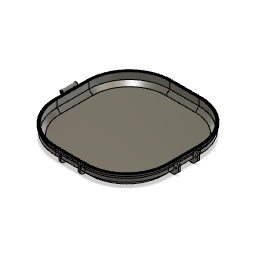
BoxFilament_Remix (Autodesk Fusion 360 archive; units mm, degrees)
design "BoxFilament_Lid_VII_v6"
Autodesk Fusion 360 part; units mm, degrees
sketch "Sketch1" plane through (0, 0, 0) normal (0, 1, 0) x (1, 0, 0)
  line L0 (28, -100.5) -> (-28, -100.5)
  line L1 (-98, -30.5) -> (-98, 30.5)
  line L2 (-28, 100.5) -> (28, 100.5)
  line L3 (98, 30.5) -> (98, -30.5)
  line L4 (98, -100.5) -> (-98, 100.5) construction
  line L5 (-98, -100.5) -> (98, 100.5) construction
  arc A0 (-28, 100.5) -> (-98, 30.5) centre (-28, 30.5) ccw
  arc A1 (98, 30.5) -> (28, 100.5) centre (28, 30.5) ccw
  arc A2 (28, -100.5) -> (98, -30.5) centre (28, -30.5) ccw
  arc A3 (-98, -30.5) -> (-28, -100.5) centre (-28, -30.5) ccw
  line L6 (15, 100.5) -> (15, -100.5)
  line L7 (-15, 100.5) -> (-15, -100.5)
  line L8 (-98, 15) -> (98, 15)
  line L9 (-98, -15) -> (98, -15)
  line L10 (0, 0) -> (0, -36) construction
  circle A4 centre (0, -36) radius 1.85
  circle A5 centre (36, 0) radius 1.85
  circle A6 centre (0, 36) radius 1.85
  circle A7 centre (-36, 0) radius 1.85
  dimension "d6" = 201
  dimension "d7" = 196
  dimension "d8" = 70
  dimension "d9" = 70
  dimension "d10" = 70
  dimension "d11" = 70
  dimension "d150" = 15
  dimension "d151" = 15
  dimension "d176" = 15
  dimension "d177" = 15
  dimension "d218" = 36
  dimension "d219" = 3.7
  dimension "d221" = 360
  constraint horizontal L0
  constraint perpendicular L0 L1
  constraint parallel L0 L2
  constraint parallel L1 L3
  constraint coincident L4 L10.start
  constraint coincident L5 L10.start
  constraint coincident L10.start origin
  constraint coincident L4.end L2
  constraint coincident L4.end L1
  constraint tangent L2 A0
  constraint tangent L1 A0
  constraint coincident L5.end L2
  constraint coincident L5.end L3
  constraint tangent L2 A1
  constraint tangent L3 A1
  constraint coincident L4.start L3
  constraint coincident L4.start L0
  constraint tangent L3 A2
  constraint tangent L0 A2
  constraint coincident L5.start L0
  constraint coincident L5.start L1
  constraint tangent L0 A3
  constraint tangent L1 A3
  constraint coincident L2 L6.start
  constraint coincident L0 L6.end
  constraint vertical L6
  constraint coincident L2 L7.start
  constraint coincident L0 L7.end
  constraint vertical L7
  constraint coincident L1 L8.start
  constraint coincident L3 L8.end
  constraint coincident L1 L9.start
  constraint coincident L3 L9.end
  constraint horizontal L8
  constraint horizontal L9
  constraint vertical L10
  constraint coincident L10.end A4.centre
  measures "d6" distance of L0 L2
  measures "d7" distance of L1 L3
  measures "d8" radius of A0
  measures "d9" radius of A1
  measures "d10" radius of A2
  measures "d11" radius of A3
  measures "d150" distance of L10.start L7
  measures "d151" distance of L10.start L6
  measures "d176" distance of L10.start L8
  measures "d177" distance of L10.start L9
  measures "d218" distance of L10.start L10.end
  measures "d219" diameter of A4
sketch "Sketch2" plane through (0, 0, 0) normal (0, 0, 1) x (1, 0, 0)
  line L0 (0, 0) -> (98, 0)
  line L1 (98, 0) -> (98, 2.4)
  line L2 (105, 9.4) -> (105, 22.4)
  line L3 (105, 22.4) -> (106.23, 22.4)
  line L4 (106.23, 22.4) -> (106.23, 20.4)
  line L5 (106.23, 20.4) -> (108.03, 20.4)
  line L6 (108.03, 20.4) -> (108.03, 22.4)
  line L7 (108.03, 22.4) -> (109.26, 22.4)
  line L8 (109.26, 22.4) -> (109.26, 19.4)
  line L9 (108.1865, 0) -> (98, 0)
  line L10 (109.26, 19.4) -> (107.4, 19.4)
  line L11 (107.4, 19.4) -> (107.4, 15)
  line L12 (107.4, 15) -> (107.4, 8.4059)
  line L13 (107.4, 15) -> (109.26, 19.4)
  line L14 (105, 9.4) -> (98, 2.4)
  line L15 (98.9941, 0) -> (107.4, 8.4059)
  line L16 (108.1865, 0) -> (116.26, 8.0735)
  line L17 (109.26, 22.4) -> (111.26, 22.4)
  line L18 (116.26, 17.4) -> (116.26, 8.0735)
  arc A0 (116.26, 17.4) -> (111.26, 22.4) centre (111.26, 17.4) ccw
  circle A1 centre (111.76, 12.4) radius 1.425
  line L19 (0, 0) -> (0, 60)
  line L20 (-116.26, 17.4) -> (-116.26, 8.0735)
  line L21 (-106.23, 22.4) -> (-106.23, 20.4)
  line L22 (-107.4, 15) -> (-109.26, 19.4)
  line L23 (-105, 9.4) -> (-105, 22.4)
  line L24 (-98, 0) -> (-98, 2.4)
  line L25 (-106.23, 20.4) -> (-108.03, 20.4)
  line L26 (-98.9941, 0) -> (-107.4, 8.4059)
  line L27 (-107.4, 15) -> (-107.4, 8.4059)
  line L28 (-105, 9.4) -> (-98, 2.4)
  line L29 (-109.26, 22.4) -> (-109.26, 19.4)
  line L30 (-108.1865, 0) -> (-116.26, 8.0735)
  line L31 (-107.4, 19.4) -> (-107.4, 15)
  line L32 (-108.03, 22.4) -> (-109.26, 22.4)
  line L33 (-108.03, 20.4) -> (-108.03, 22.4)
  line L34 (-108.1865, 0) -> (-98, 0)
  line L35 (-109.26, 19.4) -> (-107.4, 19.4)
  line L36 (-105, 22.4) -> (-106.23, 22.4)
  line L37 (107.4, 19.4) -> (105, 19.4)
  line L38 (-107.4, 19.4) -> (-105, 19.4)
  circle A2 centre (-112.86, 22.4) radius 1.425
  circle A3 centre (-112.86, 22.4) radius 3.4
  line L39 (-116.26, 22.4) -> (-116.26, 17.4)
  line L40 (-109.26, 22.4) -> (-109.46, 22.4)
  line L41 (-115.2642, 19.9958) -> (-105, 9.7317)
  line L42 (-115.2642, 19.9958) -> (-39.091, 19.9958) construction
  line L43 (-109.26, 22.4) -> (-112.86, 22.4)
  line L44 (106.23, 22.4) -> (108.03, 22.4)
  line L45 (106.38, 22.4) -> (106.38, 20.4)
  line L46 (107.88, 22.4) -> (107.88, 20.4)
  line L47 (107.13, 22.4) -> (107.13, 23.3002)
  line L48 (106.38, 22.4) -> (107.13, 23.3002)
  line L49 (107.13, 23.3002) -> (107.88, 22.4)
  line L50 (107.13, 23.3002) -> (107.33, 23.3002)
  line L51 (107.33, 23.3002) -> (107.33, 23.0602)
  line L52 (107.13, 23.3002) -> (106.93, 23.3002)
  line L53 (106.93, 23.3002) -> (106.93, 23.0602)
  point P0 (116.26, 22.4)
  point P1 (-116.26, 22.4)
  dimension "d12" = 98
  dimension "d13" = 2.4
  dimension "d15" = 1.23
  dimension "d16" = 2
  dimension "d17" = 1.8
  dimension "d18" = 2
  dimension "d20" = 3
  dimension "d23" = 4.4
  dimension "d26" = 2.4
  dimension "d27" = 7
  dimension "d28" = 7
  dimension "d29" = 22.4
  dimension "d30" = 6.5
  dimension "d61" = 7
  dimension "d62" = 5
  dimension "d63" = 2.85
  dimension "d64" = 10
  dimension "d65" = 4.5
  dimension "d129" = 1.23
  dimension "d131" = 2.4
  dimension "d137" = 2.85
  dimension "d138" = 3.6
  dimension "d139" = 6.8
  dimension "d140" = 45
  dimension "d248" = 0.15
  dimension "d249" = 0.15
  dimension "d250" = 79.6
  dimension "d251" = 0.24
  dimension "d252" = 0.24
  constraint coincident L0.start L19.start
  constraint horizontal L0
  constraint perpendicular L0 L1
  constraint perpendicular L2 L3
  constraint perpendicular L3 L4
  constraint perpendicular L4 L5
  constraint perpendicular L5 L6
  constraint perpendicular L6 L7
  constraint perpendicular L7 L8
  constraint perpendicular L1 L9
  constraint perpendicular L8 L10
  constraint perpendicular L10 L11
  constraint perpendicular L9 L12
  constraint coincident L9 L15.start
  constraint vertical L2
  constraint perpendicular L8 L17
  constraint perpendicular L7 L18
  constraint coincident P0 L17
  constraint coincident P0 L18
  constraint tangent L17 A0
  constraint tangent L18 A0
  constraint perpendicular L0 L19
  constraint symmetric L0.end L19 L24.start
  constraint symmetric L1.end L19 L24.end
  constraint symmetric L2.end L19 L23.end
  constraint symmetric L3.end L19 L21.start
  constraint symmetric L4.end L19 L21.end
  constraint symmetric L5.end L19 L25.end
  constraint symmetric L6.end L19 L32.start
  constraint symmetric L7.end L19 L29.start
  constraint symmetric L8.end L19 L22.end
  constraint symmetric L10.end L19 L31.start
  constraint symmetric L11.end L19 L22.start
  constraint symmetric L2.start L19 L23.start
  constraint symmetric L15.start L19 L26.start
  constraint symmetric L12.end L19 L26.end
  constraint symmetric L9.start L19 L30.start
  constraint symmetric P0 L19 P1
  constraint symmetric L16.end L19 L20.end
  constraint symmetric L18.start L19 L20.start
  constraint coincident L2 L37.end
  constraint perpendicular L2 L37
  constraint coincident L23 L38.end
  constraint perpendicular L23 L38
  constraint concentric A2 A3
  constraint coincident P1 L39.start
  constraint coincident A3 L40.end
  constraint horizontal L42
  constraint coincident A3 L41.start
  constraint tangent A3 L41
  constraint coincident L23 L41.end
  constraint horizontal L40
  constraint coincident A2.centre A3.centre
  constraint perpendicular L29 L43
  constraint coincident L44 L45.start
  constraint coincident L5 L45.end
  constraint perpendicular L5 L45
  constraint coincident L44 L46.start
  constraint coincident L5 L46.end
  constraint perpendicular L5 L46
  constraint midpoint L44 L47.start
  constraint perpendicular L44 L47
  constraint perpendicular L47 L50
  constraint coincident L49 L51.end
  constraint perpendicular L50 L51
  constraint perpendicular L47 L52
  constraint coincident L48 L53.end
  constraint perpendicular L52 L53
  measures "d12" distance of L0.start L0.end
  measures "d13" distance of L0.end L1.end
  measures "d15" distance of L2.end L3.end
  measures "d16" distance of L3.end L4.end
  measures "d17" distance of L4.end L5.end
  measures "d18" distance of L5.end L6.end
  measures "d20" distance of L7.end L8.end
  measures "d23" distance of L10.end L11.end
  measures "d26" distance of L14 L15
  measures "d27" vertical distance of L1.end L2.start
  measures "d28" horizontal distance of L1.end L2.start
  measures "d29" distance of L0.end L7
  measures "d30" distance of L15 L16
  measures "d61" distance of L7.end P0
  measures "d62" radius of A0
  measures "d63" diameter of A1
  measures "d64" distance of L17 A1.centre
  measures "d65" distance of L18 A1.centre
  measures "d129" distance of L6 L8
  measures "d131" distance of L2 L12
  measures "d137" diameter of A2
  measures "d138" distance of L29.start A2.centre
  measures "d139" diameter of A3
  measures "d140" angle of L41 L42
  measures "d248" distance of L6 L46
  measures "d249" distance of L4 L45
  measures "d250" angle of L48 L49
  measures "d251" distance of L50.end L51.end
  measures "d252" distance of L52.end L53.end
extrude "Extrude1" add sketch "Sketch1" along normal blind 2.4 contours L0 L3 A2 L6 L9 | L0 L6 L7 L9 | L0 L1 A3 L7 L9 | L6 L7 L8 L9 | L3 L6 L8 L9 | L1 L7 L8 L9 | L2 L6 L7 L8 | L2 L3 A1 L6 L8 | L1 L2 A0 L7 L8 | A4 | A5 | A6 | A7 makes body 1
sweep "Sweep1" add profiles "Sketch2" path "Sketch1" along A2 L0 A3 L1 A0 L2 A1 L3 section 1 contours L1 L2 L9 L11 L12 L14 L15 L37 | L2 L3 L4 L5 L6 L7 L8 L10 L37 | L10 L11 L13 | L4 L5 L44 L45 | L44 L47 L48 | L5 L44 L45 L46 | L5 L6 L44 L46 | L44 L47 L49 | L48 L52 L53 | L49 L50 L51 bodies 1
ref_plane "WorkPlane2" through (-18.4, 0, 0) normal (1, 0, 0) x (0, 1, 0)
sketch "Sketch4" plane through (-18.4, 0, 0) normal (1, 0, 0) x (0, 0, -1)
  line L0 (0, 0) -> (-100.5, 0)
  line L1 (-100.5, 0) -> (-100.5, 2.4)
  line L2 (-100.5, 2.4) -> (-107.5, 2.4)
  line L3 (-107.5, 2.4) -> (-107.5, 9.4)
  line L4 (-107.5, 9.4) -> (-100.5, 2.4)
  line L5 (-107.5, 2.4) -> (-107.5, 5)
  line L6 (-107.5, 2.4) -> (-107.5, 19.4)
  line L7 (-107.5, 19.4) -> (-111.76, 19.4)
  line L8 (-111.76, 19.4) -> (-111.76, 4.4676)
  line L9 (-107.2924, 0) -> (-100.5, 0)
  line L10 (-107.2924, 0) -> (-111.76, 4.4676)
  line L11 (0, 0) -> (0, 70)
  line L12 (107.2924, 0) -> (111.76, 4.4676)
  line L13 (107.2924, 0) -> (100.5, 0)
  line L14 (107.5, 2.4) -> (107.5, 5)
  line L15 (107.5, 2.4) -> (107.5, 19.4)
  line L16 (107.5, 9.4) -> (100.5, 2.4)
  line L17 (107.5, 2.4) -> (107.5, 9.4)
  line L18 (107.5, 19.4) -> (111.76, 19.4)
  line L19 (111.76, 19.4) -> (111.76, 4.4676)
  line L20 (100.5, 0) -> (100.5, 2.4)
  line L21 (100.5, 2.4) -> (107.5, 2.4)
  dimension "d47" = 100.5
  dimension "d48" = 2.4
  dimension "d49" = 7
  dimension "d50" = 7
  dimension "d52" = 4.26
  dimension "d53" = 6.5
  dimension "d56" = 19.4
  constraint coincident L0.start L11.start
  constraint horizontal L0
  constraint perpendicular L0 L1
  constraint perpendicular L1 L2
  constraint perpendicular L2 L3
  constraint coincident L3 L5.end
  constraint perpendicular L2 L6
  constraint perpendicular L6 L7
  constraint perpendicular L7 L8
  constraint perpendicular L1 L9
  constraint perpendicular L0 L11
  constraint symmetric L0.end L11 L13.end
  constraint symmetric L1.end L11 L16.end
  constraint symmetric L2.end L11 L14.start
  constraint symmetric L3.end L11 L16.start
  constraint symmetric L5.end L11 L14.end
  constraint symmetric L6.end L11 L15.end
  constraint symmetric L7.end L11 L18.end
  constraint symmetric L8.end L11 L12.end
  constraint symmetric L9.start L11 L12.start
  measures "d47" distance of L0.start L0.end
  measures "d48" distance of L0.end L1.end
  measures "d49" distance of L1.end L2.end
  measures "d50" distance of L2.end L3.end
  measures "d52" distance of L6.end L7.end
  measures "d53" distance of L4 L10
  measures "d56" distance of L7 L9
extrude "Extrude2" add sketch "Sketch4" along normal mid plane 3.2 bodies 1
ref_plane "WorkPlane3" through (18.4, 0, 0) normal (1, 0, 0) x (0, 1, 0)
sketch "Sketch5" plane through (18.4, 0, 0) normal (1, 0, 0) x (0, 0, -1)
  line L0 (-107.5, 2.4) -> (-107.5, 19.4)
  line L1 (-107.5, 9.4) -> (-100.5, 2.4)
  line L2 (-100.5, 2.4) -> (-107.5, 2.4)
  line L3 (-100.5, 0) -> (-100.5, 2.4)
  line L4 (-107.2924, 0) -> (-100.5, 0)
  line L5 (-107.2924, 0) -> (-111.76, 4.4676)
  line L6 (-111.76, 19.4) -> (-111.76, 4.4676)
  line L7 (-107.5, 19.4) -> (-111.76, 19.4)
  line L8 (107.5, 19.4) -> (111.76, 19.4)
  line L9 (111.76, 19.4) -> (111.76, 4.4676)
  line L10 (107.5, 2.4) -> (107.5, 19.4)
  line L11 (107.5, 9.4) -> (100.5, 2.4)
  line L12 (100.5, 2.4) -> (107.5, 2.4)
  line L13 (107.2924, 0) -> (111.76, 4.4676)
  line L14 (100.5, 0) -> (100.5, 2.4)
  line L15 (107.2924, 0) -> (100.5, 0)
extrude "Extrude3" add sketch "Sketch5" along normal mid plane 3.2 bodies 1
ref_plane "WorkPlane4" through (0, 0, -16.8) normal (0, 0, 1) x (1, 0, 0)
sketch "Sketch6" plane through (0, 0, -16.8) normal (0, 0, 1) x (1, 0, 0)
  line L0 (109.26, 22.4) -> (111.26, 22.4)
  line L1 (116.26, 17.4) -> (116.26, 8.0735)
  arc A0 (116.26, 17.4) -> (111.26, 22.4) centre (111.26, 17.4) ccw
  line L2 (108.1865, 0) -> (116.26, 8.0735)
  line L3 (108.1865, 0) -> (98, 0)
  line L4 (98, 0) -> (98, 2.4)
  line L5 (105, 9.4) -> (98, 2.4)
  line L6 (105, 9.4) -> (105, 22.4)
  line L7 (107.4, 19.4) -> (105, 19.4)
  line L8 (109.26, 19.4) -> (107.4, 19.4)
  line L9 (109.26, 22.4) -> (109.26, 19.4)
  line L10 (-105, 9.4) -> (-105, 22.4)
  line L11 (-107.4, 19.4) -> (-105, 19.4)
  line L12 (-109.26, 19.4) -> (-107.4, 19.4)
  line L13 (-109.26, 22.4) -> (-109.26, 19.4)
  line L14 (-116.26, 17.4) -> (-116.26, 8.0735)
  line L15 (-108.1865, 0) -> (-116.26, 8.0735)
  line L16 (-108.1865, 0) -> (-98, 0)
  line L17 (-98, 0) -> (-98, 2.4)
  line L18 (-105, 9.4) -> (-98, 2.4)
  circle A1 centre (111.76, 12.4) radius 1.425
  line L19 (-116.26, 22.4) -> (-116.26, 17.4)
  circle A2 centre (-112.86, 22.4) radius 3.4
  circle A3 centre (-112.86, 22.4) radius 1.425
  line L20 (-109.26, 22.4) -> (-109.46, 22.4)
  line L21 (-115.2642, 19.9958) -> (-105, 9.7317)
  point P0 (116.26, 22.4)
  point P1 (111.76, 12.4)
extrude "Extrude10" add sketch "Sketch6" against normal blind 3.2 contours L0 L1 A0 L2 L3 L4 L5 L6 L7 L8 L9 bodies 1
ref_plane "WorkPlane5" through (0, 0, 16.8) normal (0, 0, 1) x (1, 0, 0)
sketch "Sketch7" plane through (0, 0, 16.8) normal (0, 0, 1) x (1, 0, 0)
  line L0 (-98, 0) -> (-98, 2.4)
  line L1 (-105, 9.4) -> (-98, 2.4)
  line L2 (-105, 9.4) -> (-105, 22.4)
  line L3 (-107.4, 19.4) -> (-105, 19.4)
  line L4 (-109.26, 19.4) -> (-107.4, 19.4)
  line L5 (-109.26, 22.4) -> (-109.26, 19.4)
  line L6 (-116.26, 17.4) -> (-116.26, 8.0735)
  line L7 (-108.1865, 0) -> (-116.26, 8.0735)
  line L8 (-108.1865, 0) -> (-98, 0)
  line L9 (98, 0) -> (98, 2.4)
  line L10 (105, 9.4) -> (98, 2.4)
  line L11 (105, 9.4) -> (105, 22.4)
  line L12 (107.4, 19.4) -> (105, 19.4)
  line L13 (109.26, 19.4) -> (107.4, 19.4)
  line L14 (109.26, 22.4) -> (109.26, 19.4)
  line L15 (109.26, 22.4) -> (111.26, 22.4)
  arc A0 (116.26, 17.4) -> (111.26, 22.4) centre (111.26, 17.4) ccw
  line L16 (116.26, 17.4) -> (116.26, 8.0735)
  line L17 (108.1865, 0) -> (116.26, 8.0735)
  line L18 (108.1865, 0) -> (98, 0)
  circle A1 centre (111.76, 12.4) radius 1.425
  line L19 (-116.26, 22.4) -> (-116.26, 17.4)
  circle A2 centre (-112.86, 22.4) radius 3.4
  line L20 (-109.26, 22.4) -> (-109.46, 22.4)
  circle A3 centre (-112.86, 22.4) radius 1.425
  line L21 (-115.2642, 19.9958) -> (-105, 9.7317)
extrude "Extrude11" add sketch "Sketch7" along normal blind 3.2 contours L9 L10 L11 L12 L13 L14 L15 A0 L16 L17 L18 bodies 1
sketch "Sketch16" plane through (0, 0, 0) normal (0, 0, 1) x (1, 0, 0)
  circle A0 centre (-112.86, 22.4) radius 3.4
  line L0 (-109.26, 22.4) -> (-109.26, 19.4)
  line L1 (-109.26, 19.4) -> (-107.4, 19.4)
  line L2 (-107.4, 19.4) -> (-105, 19.4)
  line L3 (-105, 9.4) -> (-105, 22.4)
  line L4 (-105, 9.4) -> (-98, 2.4)
  line L5 (-98, 0) -> (-98, 2.4)
  line L6 (-108.1865, 0) -> (-98, 0)
  line L7 (-108.1865, 0) -> (-116.26, 8.0735)
  line L8 (-115.2642, 19.9958) -> (-105, 9.7317)
  line L9 (-116.26, 17.4) -> (-116.26, 8.0735)
  line L10 (-116.26, 22.4) -> (-116.26, 17.4)
  circle A1 centre (-112.86, 22.4) radius 1.425
  line L11 (-109.26, 22.4) -> (-109.46, 22.4)
extrude "Extrude33" add sketch "Sketch16" along normal mid plane 27.4 contours A0 | A0 L0 L1 L2 L3 L8 L11 bodies 1
extrude "Extrude34" add sketch "Sketch16" along normal mid plane 3.2 contours A0 L3 L4 L5 L6 L7 L8 L9 L10 bodies 1
copy_body "Body->Comp1" bodies 1 removing the originals makes body 2 in component "Spool lid"
component "Spool lid" placed x (1, 0, 0) y (0, 1, 0) z (0, 0, 1) at (0, 0, 0)
equation "width = 210 mm" comment "Min=60 (Outer dimension + 22.4mm)"
equation "lengh = 215 mm" comment "Min=120 (Outer dimension + 8.4mm)"
equation "hight = 20 mm" comment "Min=20"
equation "d6 = lengh - 14 mm"
equation "d7 = width - 14 mm"
equation "d8 = rcorner"
equation "d9 = rcorner"
equation "d10 = rcorner"
equation "d11 = rcorner"
equation "d12 = width * 0.5 - 7 mm"
equation "d13 = tbox"
equation "d26 = tbox"
equation "d29 = hight + tbox"
equation "d31 = tbox"
equation "d46 = ( -wrib + trib ) * 0.5"
equation "d47 = lengh * 0.5 - 7 mm"
equation "d48 = tbox"
equation "d54 = trib / 2"
equation "d56 = hight - 3 mm + tbox"
equation "d57 = ( wrib - trib ) * 0.5"
equation "d58 = trib / 2"
equation "d60 = -wrib * 0.5 + trib"
equation "d63 = screwhole"
equation "d68 = wrib - 2 * trib"
equation "d81 = -trib"
equation "d83 = trib"
equation "screwhole = 2.85 mm" comment "For M3 screws"
equation "rcorner = 70 mm" comment "Min=1 Max=10"
equation "d131 = tbox"
equation "tbox = 2.4 mm" comment "Min=2 Max=4.2 Box thickness"
equation "trib = 3.2 mm" comment "Min=2.4 Max=3.6 Rib thickness"
equation "d137 = screwhole"
equation "wrib = 40 mm" comment "Width between two ribs"
equation "d244 = ( wrib - trib * 2 - 6 mm - 0.2 mm ) / 2"
equation "d246 = trib / 2"
named bodies: "Box Waterproof", "BoxW"
